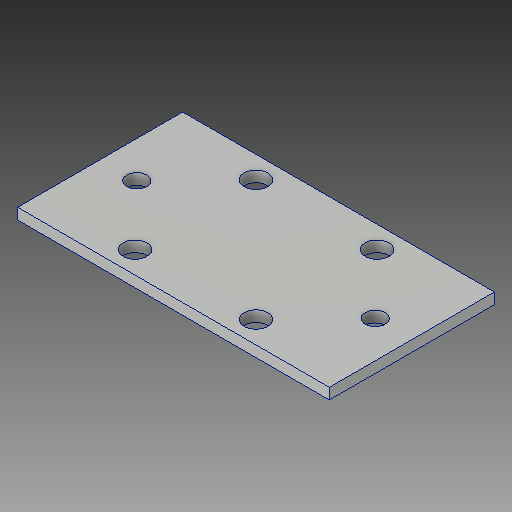
# Autodesk Inventor part: Pneumatic Bottom Plate
Saved by Autodesk Inventor 2019.4 (Build 234330000, 330)
## iProperties
Created: 2020-01-26
Part Number: Pneumatic Bottom Plate
Material: Aluminum 6061
Document SubType Name: Modeling
Designer: Mark
Mass: 29.5225 g
Surface Area: 84.1822 cm^2
Volume: 10.9343 cm^3
Density: 2.7 g/cm^3
Appearance: Aluminum - Flat
Author: Mark
Autodesk Inventor part; units mm, degrees
ref_plane "YZ Plane" through (0, 0, 0) normal (1, 0, 0) x (0, 1, 0)
ref_plane "XZ Plane" through (0, 0, 0) normal (0, 1, 0) x (-1, 0, 0)
ref_plane "XY Plane" through (0, 0, 0) normal (0, 0, 1) x (1, 0, 0)
sketch "Sketch1" plane through (0, 0, 0) normal (0, 1, 0) x (-1, 0, 0)
  line L0 (-42.5, 22.5) -> (42.5, 22.5)
  line L1 (42.5, 22.5) -> (42.5, -22.5)
  line L2 (42.5, -22.5) -> (-42.5, -22.5)
  line L3 (-42.5, -22.5) -> (-42.5, 22.5)
  line L4 (-42.5, 22.5) -> (42.5, -22.5) construction
  line L5 (42.5, 22.5) -> (-42.5, -22.5) construction
  line L6 (-22.5, 22.5) -> (22.5, 22.5)
  line L7 (22.5, 22.5) -> (22.5, -22.5)
  line L8 (22.5, -22.5) -> (-22.5, -22.5)
  line L9 (-22.5, -22.5) -> (-22.5, 22.5)
  line L10 (-22.5, 22.5) -> (22.5, -22.5) construction
  line L11 (22.5, 22.5) -> (-22.5, -22.5) construction
  circle A0 centre (32.5, 0) radius 2.75
  circle A1 centre (-32.5, 0) radius 2.75
  line L12 (-16.5, 16.5) -> (16.5, 16.5) construction
  line L13 (16.5, 16.5) -> (16.5, -16.5) construction
  line L14 (16.5, -16.5) -> (-16.5, -16.5) construction
  line L15 (-16.5, -16.5) -> (-16.5, 16.5) construction
  line L16 (-16.5, 16.5) -> (16.5, -16.5) construction
  line L17 (16.5, 16.5) -> (-16.5, -16.5) construction
  circle A2 centre (16.5, 16.5) radius 3.25
  circle A3 centre (16.5, -16.5) radius 3.25
  circle A4 centre (-16.5, 16.5) radius 3.25
  circle A5 centre (-16.5, -16.5) radius 3.25
  circle A6 centre (0, 0) radius 16.5
  dimension "d0" = 85
  dimension "d1" = 45
  dimension "d2" = 45
  dimension "d3" = 45
  dimension "d4" = 5.5
  dimension "d5" = 5.5
  dimension "d6" = 10
  dimension "d7" = 22.5
  dimension "d8" = 10
  dimension "d9" = 22.5
  dimension "d10" = 33
  dimension "d11" = 33
  dimension "d12" = 6.5
  dimension "d13" = 6.5
  dimension "d14" = 6.5
  dimension "d15" = 6.5
  dimension "d16" = 33
  constraints: 36 end point, 7 centre point, 6 midpoint, 6 parallel, 5 coincident, 3 horizontal, 3 perpendicular
  measures "d0" distance of L1.end L2.end
  measures "d1" distance of L0.end L1.end
  measures "d2" distance of L7.end L8.end
  measures "d3" distance of L6.end L7.end
  measures "d4" diameter of A0
  measures "d5" diameter of A1
  measures "d6" distance from line of L3 A1.centre
  measures "d7" distance from line of L2 A1.centre
  measures "d8" distance from line of A0.centre L1
  measures "d9" distance from line of L2 A0.centre
  measures "d10" distance of L13.end L14.end
  measures "d11" distance of L12.end L13.end
  measures "d12" diameter of A2
  measures "d13" diameter of A3
  measures "d14" diameter of A4
  measures "d15" diameter of A5
  measures "d16" diameter of A6
extrude "Extrusion1" add sketch "Sketch1" along normal blind 3 contours L0 L9 L2 L3 | L0 L7 L2 L9 | L0 L1 L2 L7 | A6
body "Solid1"
